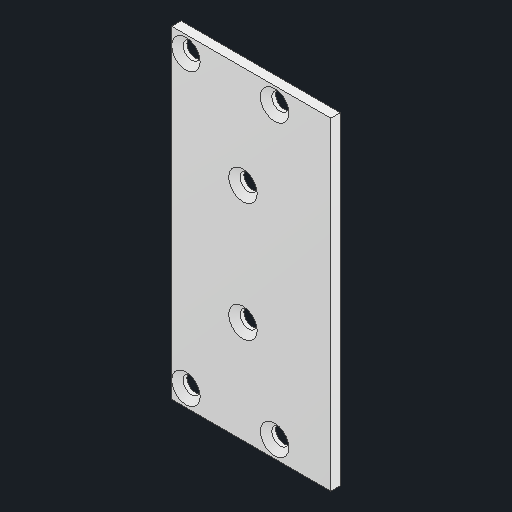
# Autodesk Inventor part: back
Saved by Autodesk Inventor 2023 (Build 270158000, 158)
## iProperties
Created: 2024-04-30
Part Number: back
Material: ABS Plastic
Document SubType Name: Modeling
Designer: szymo
Density: 1.06 g/cm^3
Appearance: Smooth - White
Mass: 3.64846 g
Surface Area: 54.9656 cm^2
Volume: 3.44195 cm^3
Author: szymo
Autodesk Inventor part; units mm, degrees
ref_plane "YZ Plane" through (0, 0, 0) normal (1, 0, 0) x (0, 1, 0)
ref_plane "XZ Plane" through (0, 0, 0) normal (0, 1, 0) x (-1, 0, 0)
ref_plane "Work Plane1" through (0, 0, 0) normal (0, 0, 1) x (1, 0, 0)
sketch "Sketch1" plane through (0, 0, 0) normal (0, 0, 1) x (1, 0, 0)
  line L0 (0, 0) -> (0, 68) projected
  line L1 (-3.5, 0) -> (-3.5, 68) projected
  line L2 (0, 0) -> (-3.5, 0) projected
  line L3 (-3.5, 7) -> (-3.5, 0) projected
  line L4 (-3.5, 7) -> (-33.5, 7) projected
  line L5 (-33.5, 7) -> (-33.5, 0) projected
  line L6 (-6.5, 0) -> (-33.5, 0) projected
  line L7 (-3.5, 0) -> (-6.5, 0) projected
  line L8 (-33.5, 19) -> (-33.5, 24) projected
  line L9 (-33.5, 19) -> (-3.5, 19) projected
  line L10 (-3.5, 19) -> (-3.5, 24) projected
  line L11 (-3.5, 24) -> (-33.5, 24) projected
  line L12 (-33.5, 49) -> (-33.5, 44) projected
  line L13 (-3.5, 44) -> (-33.5, 44) projected
  line L14 (-3.5, 49) -> (-3.5, 44) projected
  line L15 (-33.5, 49) -> (-3.5, 49) projected
  line L16 (-3.5, 61) -> (-3.5, 68) projected
  line L17 (-3.5, 68) -> (-6.5, 68) projected
  line L18 (-6.5, 68) -> (-33.5, 68) projected
  line L19 (-33.5, 61) -> (-33.5, 68) projected
  line L20 (-3.5, 61) -> (-33.5, 61) projected
  line L21 (-34.5, 123) -> (10.5, 123) projected
  line L22 (10.5, -55) -> (-34.5, -55) projected
  line L23 (-33.5, 123) -> (-33.5, -55.3182)
  circle A0 centre (-30.5, 64.5) radius 2.3 projected
  circle A1 centre (-11.8324, 64.5) radius 2.3 projected
  circle A2 centre (-18.5, 21.5) radius 2.3 projected
  circle A3 centre (-18.5, 46.5) radius 2.3 projected
  line L24 (0, -55) -> (0, 123)
  line L25 (0, 68) -> (-3.5, 68) projected
  point P0 (-33.5, -55)
  dimension "d10" = 0
  dimension "d41" = 0
  constraints: 4 end point, 3 point on line, 2 perpendicular
  measures "d10" distance between parallel lines of L0 L24
  measures "d41" distance between parallel lines of L23 L8
extrude "Extrusion1" add sketch "Sketch1" along normal blind 2 contours L2 L1 L25 L0 | L7 L6 L5 L4 L1 | L1 L20 L19 L18 L17 | L4 L23 L9 L1 | L1 L15 L23 L20 | L9 L8 L11 L1 | L1 L13 L12 L15 | L11 L23 L13 L1 | A0 | A1 | A2 | A3
sketch "Sketch2" plane through (0, 0, 2) normal (0, 0, 1) x (1, 0, 0)
  circle A0 centre (-30.5, 3.5) radius 2.3 projected
  circle A1 centre (-11.8324, 3.5) radius 2.3 projected
  line L0 (-3.5, 7) -> (-3.5, 0) projected
  line L1 (-3.5, 7) -> (-33.5, 7) projected
  line L2 (-33.5, 7) -> (-33.5, 0) projected
  line L3 (-6.5, 0) -> (-33.5, 0) projected
  line L4 (-3.5, 0) -> (-6.5, 0) projected
  circle A2 centre (-18.5, 46.5) radius 2.3 projected
  line L5 (-33.5, 49) -> (-33.5, 44) projected
  line L6 (-3.5, 44) -> (-33.5, 44) projected
  line L7 (-3.5, 49) -> (-3.5, 44) projected
  line L8 (-33.5, 49) -> (-3.5, 49) projected
  circle A3 centre (-18.5, 21.5) radius 2.3 projected
  line L9 (-33.5, 19) -> (-33.5, 24) projected
  line L10 (-33.5, 19) -> (-3.5, 19) projected
  line L11 (-3.5, 19) -> (-3.5, 24) projected
  line L12 (-3.5, 24) -> (-33.5, 24) projected
  circle A4 centre (-30.5, 64.5) radius 2.3 projected
  circle A5 centre (-11.8324, 64.5) radius 2.3 projected
  line L13 (-3.5, 61) -> (-3.5, 68) projected
  line L14 (-3.5, 68) -> (-6.5, 68) projected
  line L15 (-6.5, 68) -> (-33.5, 68) projected
  line L16 (-33.5, 61) -> (-33.5, 68) projected
  line L17 (-3.5, 61) -> (-33.5, 61) projected
  point P0 (0, 0)
  constraints: 6 coincident
hole "Hole1" at (-30.5, 3.5, 2) at (-11.8324, 3.5, 2) at (-18.5, 21.5, 2) at (-18.5, 46.5, 2) at (-30.5, 64.5, 2) at (-11.8324, 64.5, 2) direction (0, 0, -1) diameter 3.6 end through all countersink diameter 6 countersink angle 90 clearance for "Countersunk Flat Head Screw ISO 2009/7046" size "M3" standard "ISO"
sketch "Sketch3" plane through (0, 0, 0) normal (0, 0, -1) x (-1, 0, 0)
  circle A0 centre (30.5, 3.5) radius 2.3 projected
  circle A1 centre (11.8324, 3.5) radius 2.3 projected
  line L0 (3.5, 7) -> (3.5, 0) projected
  line L1 (3.5, 7) -> (33.5, 7) projected
  line L2 (33.5, 7) -> (33.5, 0) projected
  line L3 (6.5, 0) -> (33.5, 0) projected
  line L4 (3.5, 0) -> (6.5, 0) projected
  circle A2 centre (18.5, 21.5) radius 2.3 projected
  line L5 (33.5, 19) -> (33.5, 24) projected
  line L6 (33.5, 19) -> (3.5, 19) projected
  line L7 (3.5, 19) -> (3.5, 24) projected
  line L8 (3.5, 24) -> (33.5, 24) projected
  circle A3 centre (18.5, 46.5) radius 2.3 projected
  line L9 (33.5, 49) -> (33.5, 44) projected
  line L10 (3.5, 44) -> (33.5, 44) projected
  line L11 (3.5, 49) -> (3.5, 44) projected
  line L12 (33.5, 49) -> (3.5, 49) projected
  circle A4 centre (30.5, 64.5) radius 2.3 projected
  circle A5 centre (11.8324, 64.5) radius 2.3 projected
  line L13 (3.5, 61) -> (3.5, 68) projected
  line L14 (3.5, 68) -> (6.5, 68) projected
  line L15 (6.5, 68) -> (33.5, 68) projected
  line L16 (33.5, 61) -> (33.5, 68) projected
  line L17 (3.5, 61) -> (33.5, 61) projected
  line L18 (33.5, 123) -> (33.5, -55)
  line L19 (33.5, 68) -> (0, 68)
  line L20 (0, 68) -> (0, 0)
  line L21 (0, 0) -> (33.5, 0)
  line L22 (33.5, 0) -> (33.5, 68)
  line L23 (31.5, 68) -> (2, 68)
  line L24 (2, 68) -> (2, 121)
  line L25 (2, 121) -> (31.5, 121)
  line L26 (31.5, 121) -> (31.5, 68)
  line L27 (31.5, 0) -> (2, 0)
  line L28 (2, 0) -> (2, -53)
  line L29 (2, -53) -> (31.5, -53)
  line L30 (31.5, -53) -> (31.5, 0)
  line L31 (0, 123) -> (33.5, 123)
  line L32 (0, -55) -> (0, 123)
  line L33 (33.5, -55) -> (0, -55)
  line L34 (2, 68) -> (31.5, 121) construction
  line L35 (31.5, 68) -> (2, 121) construction
  line L36 (31.5, 0) -> (2, -53) construction
  line L37 (31.5, -53) -> (2, 0) construction
  line L38 (3.1445, 121) -> (31.5, 70.0562)
  line L39 (2, 118.9438) -> (30.3555, 68)
  line L40 (3.1445, 68) -> (31.5, 118.9438)
  line L41 (30.3555, 121) -> (2, 70.0562)
  line L42 (3.1445, 0) -> (31.5, -50.9438)
  line L43 (30.3555, -53) -> (2, -2.0562)
  line L44 (2, -50.9438) -> (30.3555, 0)
  line L45 (31.5, -2.0562) -> (3.1445, -53)
  line L46 (31.5, 61) -> (2, 61)
  line L47 (2, 61) -> (2, 49)
  line L48 (2, 49) -> (31.5, 49)
  line L49 (31.5, 49) -> (31.5, 61)
  line L50 (31.5, 44) -> (2, 44)
  line L51 (2, 44) -> (2, 24)
  line L52 (2, 24) -> (31.5, 24)
  line L53 (31.5, 24) -> (31.5, 44)
  line L54 (31.5, 19) -> (2, 19)
  line L55 (2, 19) -> (2, 7)
  line L56 (2, 7) -> (31.5, 7)
  line L57 (31.5, 7) -> (31.5, 19)
  line L58 (31.5, 61) -> (2, 49) construction
  line L59 (31.5, 49) -> (2, 61) construction
  line L60 (2, 44) -> (31.5, 24) construction
  line L61 (31.5, 44) -> (2, 24) construction
  line L62 (2, 19) -> (31.5, 7) construction
  line L63 (31.5, 19) -> (2, 7) construction
  line L64 (2, 50.0796) -> (28.8461, 61)
  line L65 (31.5, 59.9204) -> (4.6539, 49)
  line L66 (31.5, 50.0796) -> (4.6539, 61)
  line L67 (2, 59.9204) -> (28.8461, 49)
  line L68 (29.718, 44) -> (2, 25.2082)
  line L69 (31.5, 42.7918) -> (3.782, 24)
  line L70 (2, 42.7918) -> (29.718, 24)
  line L71 (31.5, 25.2082) -> (3.782, 44)
  line L72 (31.5, 17.9204) -> (4.6539, 7)
  line L73 (2, 8.0796) -> (28.8461, 19)
  line L74 (4.6539, 19) -> (31.5, 8.0796)
  line L75 (28.8461, 7) -> (2, 17.9204)
  line L76 (33.5, 68) -> (33.5, 0) projected
  line L77 (33.5, 3.5) -> (33.5, 0) projected
  line L78 (33.5, 64.5) -> (33.5, 3.5) projected
  line L79 (33.5, 68) -> (33.5, 64.5) projected
  line L80 (34.5, -55) -> (-10.5, -55) projected
  point P0 (16.75, -24.4438)
  point P1 (30.3555, 0)
  point P2 (3.1445, 0)
  point P3 (17.8945, -26.5)
  point P4 (16.75, -28.5562)
  point P5 (15.6055, -26.5)
  point P6 (16.75, 92.4438)
  point P7 (30.3555, 68)
  point P8 (15.6055, 94.5)
  point P9 (17.8945, 94.5)
  point P10 (16.75, 96.5562)
  point P11 (19.4039, 13)
  point P12 (28.8461, 7)
  point P13 (16.75, 11.9204)
  point P14 (4.6539, 7)
  point P15 (14.0961, 13)
  point P16 (16.75, 14.0796)
  point P17 (28.8461, 19)
  point P18 (29.718, 24)
  point P19 (16.75, 32.7918)
  point P20 (3.782, 24)
  point P21 (18.532, 34)
  point P22 (14.968, 34)
  point P23 (3.782, 44)
  point P24 (16.75, 35.2082)
  point P25 (14.0961, 55)
  point P26 (4.6539, 49)
  point P27 (16.75, 56.0796)
  point P28 (28.8461, 61)
  point P29 (19.4039, 55)
  point P30 (16.75, 53.9204)
  dimension "d11" = 2
  dimension "d12" = 2
  dimension "d13" = 2
  dimension "d14" = 2
  dimension "d15" = 2
  dimension "d16" = 2
  dimension "d17" = 1
  dimension "d18" = 1
  dimension "d19" = 1
  dimension "d20" = 1
  dimension "d21" = 1
  dimension "d22" = 1
  dimension "d23" = 1
  dimension "d24" = 1
  dimension "d27" = 2
  dimension "d28" = 2
  dimension "d29" = 1
  dimension "d30" = 1
  dimension "d31" = 1
  dimension "d32" = 1
  dimension "d33" = 1
  dimension "d34" = 1
  dimension "d35" = 1
  dimension "d36" = 1
  dimension "d37" = 1
  dimension "d38" = 1
  dimension "d39" = 1
  dimension "d40" = 1
  dimension "d42" = 0
  constraints: 116 end point, 55 point on line, 33 parallel, 6 horizontal, 6 perpendicular, 2 collinear
  measures "d11" distance between parallel lines of L18 L26
  measures "d12" distance between parallel lines of L31 L25
  measures "d13" distance between parallel lines of L24 L32
  measures "d14" distance between parallel lines of L32 L28
  measures "d15" distance between parallel lines of L18 L30
  measures "d16" distance between parallel lines of L33 L29
  measures "d17" distance between parallel lines of L36 L45
  measures "d18" distance between parallel lines of L36 L44
  measures "d19" distance between parallel lines of L37 L42
  measures "d20" distance between parallel lines of L37 L43
  measures "d21" distance between parallel lines of L38 L35
  measures "d22" distance between parallel lines of L35 L39
  measures "d23" distance between parallel lines of L34 L40
  measures "d24" distance between parallel lines of L34 L41
  measures "d27" distance between parallel lines of L47 L20
  measures "d28" distance between parallel lines of L22 L49
  measures "d29" distance between parallel lines of L58 L65
  measures "d30" distance between parallel lines of L58 L64
  measures "d31" distance between parallel lines of L59 L66
  measures "d32" distance between parallel lines of L59 L67
  measures "d33" distance between parallel lines of L61 L69
  measures "d34" distance between parallel lines of L61 L68
  measures "d35" distance between parallel lines of L60 L71
  measures "d36" distance between parallel lines of L60 L70
  measures "d37" distance between parallel lines of L63 L73
  measures "d38" distance between parallel lines of L63 L72
  measures "d39" distance between parallel lines of L62 L74
  measures "d40" distance between parallel lines of L62 L75
  measures "d42" distance between parallel lines of L76 L18
extrude "Extrusion2" cut sketch "Sketch3" against normal blind 1 contours L4 L3 L44 L42 L21 | L72 L75 L1 | L55 L75 L73 | L72 L57 L74 | L43 L44 L28 | L45 L30 L42 | L74 L6 L73 | L43 L29 L45 | L40 L39 L15 L14 L19 | L24 L39 L41 | L69 L70 L8 | L71 L69 L53 | L51 L70 L68 | L40 L26 L38 | L38 L25 L41 | L68 L71 L10 | L17 L64 L66 | L12 L65 L67 | L66 L65 L49 | L67 L64 L47
body "Solid1"
